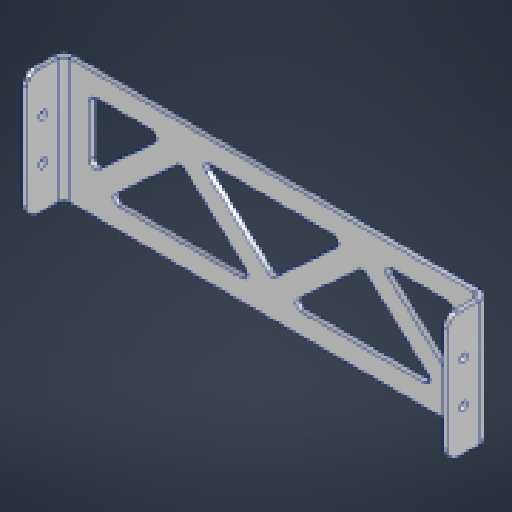
# Autodesk Inventor part: feeder_middle_brace
Saved by Autodesk Inventor 2024.3 (Build 283343000, 343)
## iProperties
Created: 2025-03-09
Part Number: feeder_middle_brace
Material: Aluminum 6061
Document SubType Name: Sheet Metal
Designer: marcu
Density: 2.7 g/cm^3
Sheet Metal Rule: Default
Appearance: Aluminum - Flat
Mass: 130.035 g
Surface Area: 356.509 cm^2
Volume: 48.1609 cm^3
Author: marcu
Autodesk Inventor part; units mm, degrees
ref_plane "YZ Plane" through (0, 0, 0) normal (1, 0, 0) x (0, 1, 0)
ref_plane "XZ Plane" through (0, 0, 0) normal (0, 1, 0) x (-1, 0, 0)
ref_plane "XY Plane" through (0, 0, 0) normal (0, 0, 1) x (1, 0, 0)
sketch "Sketch1" plane through (0, 0, 0) normal (0, 0, 1) x (1, 0, 0)
  line L0 (130.429, -38.1) -> (-130.429, -38.1)
  line L1 (-130.429, -38.1) -> (-130.429, 38.1)
  line L2 (-130.429, 38.1) -> (130.429, 38.1)
  line L3 (130.429, 38.1) -> (130.429, -38.1)
  line L4 (130.429, -38.1) -> (-130.429, 38.1) construction
  line L5 (-130.429, -38.1) -> (130.429, 38.1) construction
  point P0 (0, 0)
  dimension "d0" = 260.858
  dimension "d1" = 76.2
  measures "d0" distance of L1.end L2.end
  measures "d1" distance of L0.end L1.end
extrude "Plate1" add sketch "Sketch1" along normal blind 3.175
sketch "Sketch2" plane through (-127.254, -38.1, 0) normal (-1, 0, 0) x (0, -1, 0)
  line L0 (-76.2, 0) -> (0, 0)
  line L1 (0, 0) -> (0, 25.4)
  line L2 (0, 25.4) -> (-76.2, 25.4)
  line L3 (-76.2, 25.4) -> (-76.2, 0)
  constraints: 6 end point, 1 horizontal, 1 perpendicular, 1 vertical
edge flange "Flange1" height 25.4 angle 90 thickness 3.175 bend radius 3.175 thickness toward (-1, 0, 0) relief straight relief width 3.175 relief depth 1.5875 corner gap 3.175 corner form 0 edges at (-130.429, 0, 3.175) (130.429, 0, 3.175) wall of the first edge with corners at (-127.254, 38.1, 0) (-127.254, -38.1, 0) (-127.254, -38.1, 25.4) (-127.254, 38.1, 25.4)
bend "Bend1"
corner "Corner1"
sketch "Sketch3" plane through (-130.429, -38.1, 25.4) normal (-1, 0, 0) x (0, 0, 1)
  line L0 (0, 76.2) -> (0, 0) construction
  line L1 (-9.525, 25.4) -> (-9.525, 50.8) construction
  point P0 (-25.4, 38.1)
  point P1 (-9.525, 38.1)
  dimension "d13" = 25.4
  dimension "d14" = 9.525
  constraints: 2 end point, 1 horizontal alignment, 1 midpoint, 1 vertical, 1 vertical alignment
  measures "d13" distance of L1.end L1.start
  measures "d14" distance from line of L0 L1.start
hole "Hole1" at (-130.429, -12.7, 15.875) at (-130.429, 12.7, 15.875) direction (1, 0, 0) diameter 5.1054 end through all clearance for "Flat Head Machine Screw (82)" size "#10" standard "Ansi Unified Screw Threads"
fillet "Corner Round1" radius 6.35 4 edges at (128.8415, 38.1, 25.4) (128.8415, -38.1, 25.4) (-128.8415, 38.1, 25.4) (-128.8415, -38.1, 25.4)
sketch "Sketch5" plane through (0, 0, 0) normal (0, 0, -1) x (-1, 0, 0)
  line L0 (-124.079, 38.1) -> (-124.079, -38.1) construction
  line L1 (124.079, -38.1) -> (-124.079, -38.1) construction
  line L2 (124.079, -38.1) -> (124.079, 38.1) construction
  line L3 (-124.079, 38.1) -> (124.079, 38.1) construction
  line L4 (111.379, 25.4) -> (111.379, -25.4)
  line L5 (111.379, -25.4) -> (-111.379, -25.4)
  line L6 (-111.379, -25.4) -> (-111.379, 25.4)
  line L7 (-111.379, 25.4) -> (111.379, 25.4)
  line L8 (-111.379, -25.4) -> (-55.6895, 25.4) construction
  line L9 (-107.0995, -30.0914) -> (-51.41, 20.7086)
  line L10 (-59.969, 30.0914) -> (-115.6585, -20.7086)
  arc A0 (-115.6585, -20.7086) -> (-107.0995, -30.0914) centre (-111.379, -25.4) ccw
  arc A1 (-51.41, 20.7086) -> (-59.969, 30.0914) centre (-55.6895, 25.4) ccw
  line L11 (-55.6895, 25.4) -> (0, -25.4) construction
  line L12 (-59.969, 20.7086) -> (-4.2795, -30.0914)
  line L13 (4.2795, -20.7086) -> (-51.41, 30.0914)
  arc A2 (-51.41, 30.0914) -> (-59.969, 20.7086) centre (-55.6895, 25.4) ccw
  arc A3 (-4.2795, -30.0914) -> (4.2795, -20.7086) centre (0, -25.4) ccw
  line L14 (-111.379, 25.4) -> (0, 25.4) construction
  line L15 (0, 25.4) -> (0, -25.4) construction
  line L16 (107.0995, -30.0914) -> (51.41, 20.7086)
  line L17 (59.969, 30.0914) -> (115.6585, -20.7086)
  line L18 (59.969, 20.7086) -> (4.2795, -30.0914)
  line L19 (-4.2795, -20.7086) -> (51.41, 30.0914)
  point P0 (0, 0)
  point P1 (-83.5342, 0)
  point P2 (-27.8447, 0)
  point P3 (65.1118, 25.4)
  point P4 (111.379, -16.8049)
  point P5 (55.6895, 16.8049)
  point P6 (9.4223, -25.4)
  point P7 (101.9567, -25.4)
  point P8 (0, -16.8049)
  point P9 (46.2672, 25.4)
  point P10 (-46.2672, 25.4)
  point P11 (-9.4223, -25.4)
  point P12 (-55.6895, 16.8049)
  point P13 (-101.9567, -25.4)
  point P14 (-111.379, -16.8049)
  point P15 (-65.1118, 25.4)
  dimension "d40" = 12.7
  dimension "d41" = 12.7
  dimension "d43" = 12.7
  constraints: 36 end point, 8 point on circle, 8 symmetric about line, 8 tangent, 5 midpoint, 4 centre point, 2 parallel, 1 point on line, 1 vertical, 3 other
  measures "d40" distance between parallel lines of L3 L7
  measures "d41" diameter of A1
  measures "d43" diameter of A3
extrude "Extrusion2" cut sketch "Sketch5" against normal blind 3.175 contours L4 L17 L7 | L19 L13 L7 | L5 L18 L16 | L5 L9 L12 | L10 L6 L7
fillet "Corner Round2" radius 3.175 15 edges at (111.379, 25.4, 1.5875) (111.379, -16.8049, 1.5875) (65.1118, 25.4, 1.5875) (46.2672, 25.4, 1.5875) (101.9567, -25.4, 1.5875) (55.6895, 16.8049, 1.5875) (9.4223, -25.4, 1.5875) (0, -16.8049, 1.5875) (-9.4223, -25.4, 1.5875) (-55.6895, 16.8049, 1.5875) (-101.9567, -25.4, 1.5875) (-111.379, -16.8049, 1.5875) (-111.379, 25.4, 1.5875) (-65.1118, 25.4, 1.5875) (-46.2672, 25.4, 1.5875)
equation "\"d20\" = Thickness"
equation "\"d2\" = Thickness"
equation "\"d3\" = BendReliefWidth"
equation "\"d4\" = BendReliefDepth"
equation "\"d5\" = MinimumRemnant"
equation "\"d6\" = TransitionRadius"
equation "\"d9\" = BendRadius"
equation "\"d10\" = CornerReliefSize"
equation "\"d11\" = GapSize"
equation "\"d12\" = JacobiRadiusSize"
equation "\"BendRadius\" = Thickness"
equation "\"BendReliefWidth\" = Thickness"
equation "\"BendReliefDepth\" = 0.5 * Thickness"
equation "\"CornerReliefSize\" = 4 * Thickness"
equation "\"MinimumRemnant\" = 2 * Thickness"
equation "\"TransitionRadius\" = BendRadius"
equation "\"JacobiRadiusSize\" = BendRadius"
equation "\"GapSize\" = Thickness"
equation "\"Thickness\" = 3.175"
body "Solid1"
